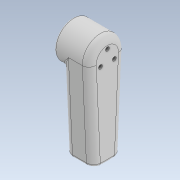
# Autodesk Inventor part: shank_link
Saved by Autodesk Inventor 2020 (Build 240168000, 168)
## iProperties
Created: 2020-12-22
Part Number: shank_link
Material: Generic
Document SubType Name: Modeling
Designer: DELL
Density: 1 g/cm^3
Appearance: Default
Author: DELL
Autodesk Inventor part; units mm, degrees
sketch "Sketch1" plane through (0, 0, 0) normal (1, 0, 0) x (0, 1, 0)
  line L0 (0, 0) -> (0, 25.2399) construction
  line L1 (0, 0) -> (0, -46.7601) construction
  line L2 (0, 0) -> (-130, 0) construction
  circle A0 centre (0, 0) radius 26
  line L3 (0, 0) -> (-13, 22.5167) construction
  line L4 (0, 0) -> (-13, -22.5167) construction
  line L5 (-1.2043, 25.9721) -> (-130, 20)
  line L6 (-1.2043, -25.9721) -> (-130, -20)
  line L7 (-130, 20) -> (-130, -20)
  circle A1 centre (0, 0) radius 11.5 construction
  circle A2 centre (11.5, 0) radius 1.65
  line L8 (0, 0) -> (26, 0) construction
  circle A3 centre (-5.75, 9.9593) radius 1.65
  circle A4 centre (-5.75, -9.9593) radius 1.65
  circle A5 centre (0, 0) radius 9.715 construction
  line L9 (0, 0) -> (5.75, 9.9593) construction
  line L10 (0, 0) -> (5.75, -9.9593) construction
  circle A6 centre (4.8575, 8.4134) radius 2
  circle A7 centre (4.8575, -8.4134) radius 2
  circle A8 centre (-9.715, 0) radius 2
  circle A9 centre (11.5, 0) radius 2.75
  circle A10 centre (-5.75, -9.9593) radius 2.75
  circle A11 centre (-5.75, 9.9593) radius 2.75
  circle A12 centre (0, 0) radius 130 construction
  arc A13 (-128.441, 20.0723) -> (-128.441, -20.0723) centre (0, 0) ccw
  line L11 (0, 0) -> (-1.2043, 25.9721) construction
  point P0 (-65, 0)
  dimension "d6" = 52
  dimension "d8" = 60
  dimension "d84" = 130
  dimension "d85" = 40
  dimension "d97" = 23
  dimension "d98" = 3.3
  dimension "d99" = 19.43
  dimension "d100" = 30
  dimension "d101" = 4
  dimension "d102" = 5.5
  dimension "d122" = 260
  dimension "d129" = 20.0723
  dimension "d130" = 128.441
  dimension "d131" = 1.559
  constraints: 24 end point, 18 point on circle, 14 centre point, 10 point on line, 7 coincident, 6 equal radius, 2 midpoint, 2 vertical, 1 horizontal, 1 perpendicular, 1 symmetric about line, 1 tangent, 3 other
  measures "d6" diameter of A0
  measures "d8" angle of L2 L3
  measures "d84" distance between parallel lines of L7 L1
  measures "d85" distance of L5.end L6.end
  measures "d97" diameter of A1
  measures "d98" diameter of A2
  measures "d99" diameter of A5
  measures "d100" angle of L0 L9
  measures "d101" diameter of A6
  measures "d102" diameter of A9
  measures "d122" diameter of A12
  measures "d129" distance from line of A12.end L2
  measures "d130" distance from line of L0 A12.end
  measures "d131" distance from line of L7 A12.end
ref_plane "Work Plane1" through (14.5, 0, 0) normal (1, 0, 0) x (0, 1, 0)
ref_plane "Work Plane2" through (-14.5, 0, 0) normal (1, 0, 0) x (0, 1, 0)
extrude "Extrusion4" add sketch "Sketch1" along normal blind 20 and the other way blind 30 contours A0 | A6 | A7 | A8 | A9 | A10 | A11
extrude "Extrusion6" cut sketch "Sketch1" against normal blind 40 from surface at 20 contours A9 | A10 | A11
extrude "Extrusion7" cut sketch "Sketch1" along normal blind 5 from surface at -30 contours A6 | A7 | A8
extrude "Extrusion9" add sketch "Sketch1" along normal mid plane 40 contours A0 L6 A13 L5
sketch "Sketch6" plane through (0, 0, 0) normal (0, 1, 0) x (-1, 0, 0)
  circle A0 centre (0, 0) radius 10
  dimension "d123" = 20
  constraints: 1 centre point, 1 coincident
  measures "d123" diameter of A0
ref_plane "Work Plane4" through (0, -130, 0) normal (0, 1, 0) x (-1, 0, 0)
extrude "Extrusion11" cut sketch "Sketch6" along normal blind 60 from surface at -130
fillet "Fillet28" radius 10 4 edges at (20, -64.8227, 23.0222) (-20, -64.8227, 23.0222) (20, -64.8227, -23.0222) (-20, -64.8227, -23.0222)
fillet "Fillet32" radius 5 3 edges at (-20, -26, 0) (-15.7828, -10.7198, -23.6873) (-16.2433, -11.5323, 23.3025)
fillet "Fillet29" radius 4 8 edges at (16.4896, -128.7947, 17.6616) (20, -130, 0) (16.4918, -128.7949, -17.6596) (0, -128.441, -20.0723) (-16.4673, -128.7921, -17.6806) (-20, -130, 0) (-16.4896, -128.7947, 17.6616) (0, -128.441, 20.0723)
fillet "Fillet31" radius 2 1 edges at (-30, -26, 0)
fillet "Fillet33" radius 2 3 edges at (-0.013, -129.6148, 10) (-0.0126, -129.6148, -10) (10, -70, 0)
body "Solid1"
